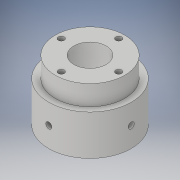
# Autodesk Inventor part: tutup_syringe
Saved by Autodesk Inventor 2019 (Build 230136000, 136)
## iProperties
Created: 2020-08-01
Part Number: tutup_syringe
Material: Generic
Document SubType Name: Modeling
Designer: Agus Prayudi
Density: 1 g/cm^3
Appearance: Default
Author: Agus Prayudi
Autodesk Inventor part; units mm, degrees
ref_plane "XZ Plane" through (0, 0, 0) normal (0, 1, 0) x (-1, 0, 0)
ref_plane "XY Plane" through (0, 0, 0) normal (0, 0, 1) x (1, 0, 0)
sketch "Sketch1" plane through (0, 0, 0) normal (0, 1, 0) x (-1, 0, 0)
  circle A0 centre (0, 0) radius 20.525
  constraints: 1 centre point, 1 coincident
extrude "Extrusion1" add sketch "Sketch1" along normal blind 30
sketch "Sketch2" plane through (0, 30, 0) normal (0, 1, 0) x (1, 0, 0)
  circle A0 centre (0, 0) radius 8.05
  dimension "d3" = 16.1
  constraints: 1 centre point, 1 coincident
  measures "d3" diameter of A0
extrude "Extrusion2" cut sketch "Sketch2" against normal blind 13
sketch "Sketch4" plane through (0, 17, 0) normal (0, 1, 0) x (1, 0, 0)
  circle A0 centre (0, 0) radius 3
  dimension "d27" = 6
  constraints: 1 centre point, 1 coincident
  measures "d27" diameter of A0
sketch "Sketch5" plane through (0, 30, 0) normal (0, 1, 0) x (1, 0, 0)
  circle A0 centre (0, 0) radius 8.05 projected
  circle A1 centre (0, 0) radius 20.525 projected
  circle A2 centre (0, 14.2875) radius 1.5
  constraints: 1 centre point
extrude "Extrusion5" cut sketch "Sketch5" against normal blind 5 contours A2
pattern_circular "Circular Pattern2" count 4 over 360 about axis through (0, 0, 0) along (0, 1, 0) of "Extrusion5"
sketch "Sketch6" plane through (0, 30, 0) normal (0, 1, 0) x (1, 0, 0)
  circle A0 centre (0, 14.2875) radius 1.5 projected
  line L0 (0, 15.7875) -> (0, 17.2875)
  circle A1 centre (0, 0) radius 17.2875
  circle A2 centre (0, 0) radius 20.525 projected
  dimension "d22" = 1.5
  constraints: 2 end point, 2 vertical alignment, 1 coincident, 1 vertical, 3 other
  measures "d22" distance of L0.start L0.end
extrude "Extrusion6" cut sketch "Sketch6" against normal blind 10 contours A2
extrude "Extrusion7" cut sketch "Sketch4" against normal blind 10
sketch "Sketch7" plane through (0, 0, 0) normal (0, -1, 0) x (1, 0, 0)
  circle A0 centre (0, 0) radius 5
  dimension "d28" = 10
  constraints: 1 centre point, 1 coincident
  measures "d28" diameter of A0
extrude "Extrusion8" cut sketch "Sketch7" against normal blind 14
sketch "Sketch8" plane through (0, 30, 0) normal (0, 1, 0) x (1, 0, 0)
  circle A0 centre (0, 0) radius 17.2875 projected
  circle A1 centre (14.2875, 0) radius 1.5 projected
  circle A2 centre (0, -14.2875) radius 1.5 projected
  circle A3 centre (-14.2875, 0) radius 1.5 projected
  circle A4 centre (0, 14.2875) radius 1.5 projected
  circle A5 centre (0, 0) radius 8.05 projected
ref_plane "Work Plane1" through (17.5, 0, 0) normal (1, 0, 0) x (0, 1, 0)
sketch "Sketch9" plane through (17.5, 0, 0) normal (1, 0, 0) x (0, 1, 0)
  circle A0 centre (10, 0) radius 1.5
  dimension "d32" = 3
  constraints: 1 centre point
  measures "d32" diameter of A0
extrude "Extrusion9" cut sketch "Sketch9" along normal blind 50 and the other way blind 50
pattern_circular "Circular Pattern3" count 4 over 360 about axis through (0, 0, 0) along (0, 1, 0) of "Extrusion9"
sketch "Sketch10" plane through (0, 0, 0) normal (0, -1, 0) x (1, 0, 0)
  line L0 (-5.6922, -5.6922) -> (-7.7428, -3.6416)
  line L1 (-7.7428, -3.6416) -> (-18.2787, -14.1775)
  line L2 (-18.2787, -14.1775) -> (-14.1775, -18.2787)
  line L3 (-14.1775, -18.2787) -> (-3.6416, -7.7428)
  line L4 (-3.6416, -7.7428) -> (-5.6922, -5.6922)
  point P0 (0, 0)
  constraints: 10 end point, 2 perpendicular, 1 collinear, 1 point on line
extrude "Extrusion10" cut sketch "Sketch10" against normal blind 10.1
body "Solid1"
